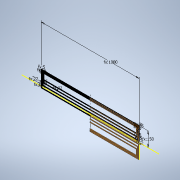
# Autodesk Inventor part: wire_half
Saved by Autodesk Inventor 2020 (Build 240168000, 168)
## iProperties
Created: 2021-01-20
Part Number: wire_half
Material: Generic
Document SubType Name: Modeling
Designer: phamv
Density: 1 g/cm^3
Appearance: Default
Author: phamv
Autodesk Inventor part; units mm, degrees
ref_plane "YZ Plane" through (0, 0, 0) normal (1, 0, 0) x (0, 1, 0)
ref_plane "XY Plane" through (0, 0, 0) normal (0, 0, 1) x (1, 0, 0)
sketch "Sketch1" plane through (0, 0, 0) normal (0, 0, 1) x (1, 0, 0)
  line L0 (0, -11) -> (500, -11)
  line L1 (500, -11) -> (500, -150)
  line L2 (500, -150) -> (-500, -150)
  line L3 (-500, -150) -> (-500, -38)
  line L4 (0, -11) -> (0, -16)
  line L5 (0, -16) -> (495, -16)
  line L6 (495, -16) -> (495, -145)
  line L7 (495, -145) -> (-495, -145)
  line L8 (-500, -38) -> (490, -38)
  line L9 (490, -38) -> (490, -140)
  line L10 (490, -140) -> (-490, -140)
  line L11 (-495, -145) -> (-495, -43)
  line L12 (-495, -43) -> (485, -43)
  line L13 (485, -43) -> (485, -135)
  line L14 (485, -135) -> (-485, -135)
  line L15 (-485, -135) -> (-485, -70)
  line L16 (-490, -140) -> (-490, -65)
  line L17 (-490, -65) -> (480, -65)
  line L18 (480, -65) -> (480, -130)
  line L19 (-485, -70) -> (475, -70)
  line L20 (475, -70) -> (475, -125)
  line L21 (-700, 0) -> (700, 0) projected
  line L22 (475, -125) -> (-480, -125)
  line L23 (480, -130) -> (-480, -130)
  line L24 (-480, -130) -> (-480, -125)
  line L25 (0, -150) -> (0, -11)
  point P0 (0, 0)
  point P1 (0, 0)
  dimension "d1" = 5
  dimension "d2" = 5
  dimension "d3" = 5
  dimension "d4" = 11
  dimension "d5" = 1000
  dimension "d6" = 500
  dimension "d7" = 5
  dimension "d8" = 5
  dimension "d9" = 5
  dimension "d10" = 5
  dimension "d11" = 22
  dimension "d12" = 5
  dimension "d13" = 5
  dimension "d14" = 5
  dimension "d15" = 5
  dimension "d16" = 5
  dimension "d17" = 5
  dimension "d19" = 22
  dimension "d20" = 5
  dimension "d82" = 150
  dimension "d88" = 5
  dimension "d89" = 5
  dimension "d90" = 5
  constraints: 50 end point, 15 perpendicular, 4 horizontal, 3 vertical, 2 parallel, 1 coincident, 1 collinear, 1 midpoint
  measures "d1" distance between parallel lines of L5 L0
  measures "d2" distance between parallel lines of L6 L1
  measures "d3" distance between parallel lines of L2 L7
  measures "d4" distance from line of L21 L0.start
  measures "d5" distance between parallel lines of L3 L1
  measures "d6" distance from line of point (0, 0) L1
  measures "d7" distance between parallel lines of L3 L11
  measures "d8" distance between parallel lines of L13 L9
  measures "d9" distance between parallel lines of L9 L6
  measures "d10" distance between parallel lines of L8 L12
  measures "d11" distance between parallel lines of L8 L5
  measures "d12" distance between parallel lines of L10 L14
  measures "d13" distance between parallel lines of L7 L10
  measures "d14" distance between parallel lines of L16 L15
  measures "d15" distance between parallel lines of L17 L19
  measures "d16" distance between parallel lines of L20 L18
  measures "d17" distance between parallel lines of L18 L13
  measures "d19" distance between parallel lines of L17 L12
  measures "d20" distance between parallel lines of L11 L16
  measures "d82" distance between parallel lines of L2 L21
  measures "d88" distance between parallel lines of L23 L22
  measures "d89" distance between parallel lines of L14 L23
  measures "d90" distance between parallel lines of L15 L24
extrude "Extrusion1" add sketch "Sketch1" along normal blind 5 contours L0 L1 L2 L25 L7 L6 L5 L4 | L25 L12 L11 L7 L2 L3 L8 | L8 L9 L10 L25 L14 L13 L12 | L25 L19 L15 L14 L10 L16 L17 | L17 L18 L23 L25 L22 L20 L19 | L25 L23 L24 L22
sketch "Sketch3" plane through (0, 0, 0) normal (0, 0, 1) x (1, 0, 0)
  line L0 (0, -16) -> (-500, -16)
  line L1 (-500, -16) -> (-500, 150)
  line L2 (-500, 150) -> (500, 150)
  line L3 (500, 150) -> (500, 11)
  line L4 (0, -11) -> (-495, -11)
  line L5 (-495, -11) -> (-495, 145)
  line L6 (-495, 145) -> (495, 145)
  line L7 (495, 145) -> (495, 16)
  line L8 (495, 16) -> (-485, 16)
  line L9 (-485, 16) -> (-485, 135)
  line L10 (500, 11) -> (-490, 11)
  line L11 (-490, 11) -> (-490, 140)
  line L12 (-485, 135) -> (485, 135)
  line L13 (-490, 140) -> (490, 140)
  line L14 (485, 135) -> (485, 43)
  line L15 (485, 43) -> (-475, 43)
  line L16 (490, 140) -> (490, 38)
  line L17 (490, 38) -> (-480, 38)
  line L18 (-475, 43) -> (-475, 125)
  line L19 (-475, 125) -> (475, 125)
  line L20 (475, 125) -> (475, 70)
  line L21 (475, 70) -> (-470, 70)
  line L22 (-480, 38) -> (-480, 130)
  line L23 (-480, 130) -> (480, 130)
  line L24 (480, 130) -> (480, 65)
  line L25 (480, 65) -> (-470, 65)
  line L26 (-470, 70) -> (-470, 65)
  line L27 (500, -150) -> (500, -11) projected
  line L28 (-700, 0) -> (700, 0) projected
  line L29 (0, 150) -> (0, -150) construction
  point P0 (0, 0)
  dimension "d58" = 5
  dimension "d59" = 5
  dimension "d60" = 5
  dimension "d61" = 5
  dimension "d62" = 5
  dimension "d64" = 5
  dimension "d65" = 5
  dimension "d66" = 5
  dimension "d67" = 5
  dimension "d68" = 1000
  dimension "d69" = 22
  dimension "d70" = 5
  dimension "d71" = 5
  dimension "d72" = 22
  dimension "d73" = 5
  dimension "d74" = 5
  dimension "d75" = 5
  dimension "d76" = 5
  dimension "d77" = 22
  dimension "d78" = 5
  dimension "d79" = 5
  dimension "d80" = 5
  dimension "d83" = 150
  dimension "d87" = 5
  constraints: 56 end point, 16 perpendicular, 4 parallel, 4 vertical, 3 horizontal, 1 collinear, 1 midpoint, 1 other
  measures "d58" distance between parallel lines of L1 L5
  measures "d59" distance between parallel lines of L2 L6
  measures "d60" distance between parallel lines of L7 L3
  measures "d61" distance between parallel lines of L13 L6
  measures "d62" distance between parallel lines of L5 L11
  measures "d64" distance between parallel lines of L10 L8
  measures "d65" distance between parallel lines of L14 L16
  measures "d66" distance between parallel lines of L13 L12
  measures "d67" distance between parallel lines of L16 L7
  measures "d68" distance between parallel lines of L1 L3
  measures "d69" distance between parallel lines of L4 L10
  measures "d70" distance between parallel lines of L11 L9
  measures "d71" distance between parallel lines of L17 L15
  measures "d72" distance between parallel lines of L8 L17
  measures "d73" distance between parallel lines of L12 L23
  measures "d74" distance between parallel lines of L9 L22
  measures "d75" distance between parallel lines of L23 L19
  measures "d76" distance between parallel lines of L24 L14
  measures "d77" distance between parallel lines of L15 L25
  measures "d78" distance between parallel lines of L24 L20
  measures "d79" distance between parallel lines of L25 L21
  measures "d80" distance between parallel lines of L22 L18
  measures "d83" distance of the line from the sketch origin of L2
  measures "d87" distance between parallel lines of L18 L26
extrude "Extrusion2" add sketch "Sketch3" along normal blind 5 fills toward (-247.5, -11.05) open curves L4 L5 L6 L7 L8 L9 L12 L14 L15 L18 L19 L20 L21 L26 L25 L24 L23 L22 L17 L16 L13 L11 L10 L3 L2 L1 L0
sketch "Sketch5" plane through (0, 0, 5) normal (0, 0, 1) x (1, 0, 0)
  line L0 (500, 150) -> (-500, 150) projected
  line L1 (-500, -150) -> (500, -150) projected
  line L2 (-500, 150) -> (0, 150)
  line L3 (0, 150) -> (0, -150)
  line L4 (0, -150) -> (-500, -150)
  line L5 (-500, -150) -> (-500, 150)
  point P0 (0, 0)
  constraints: 8 end point, 2 parallel, 1 horizontal, 1 midpoint, 1 perpendicular
extrude "Extrusion3" cut sketch "Sketch5" against normal up to surface (5 mm away)
equation "\"d1\" = wire_diameter"
equation "\"d2\" = wire_diameter"
equation "\"d3\" = wire_diameter"
equation "\"d4\" = 0.5 * distance_between_wires"
equation "\"d5\" = track_length"
equation "\"d6\" = 0.5 * track_length"
equation "\"d7\" = wire_diameter"
equation "\"d8\" = wire_diameter"
equation "\"d9\" = distance_between_wires_edge"
equation "\"d10\" = wire_diameter"
equation "\"d11\" = distance_between_wires"
equation "\"d12\" = wire_diameter"
equation "\"d13\" = distance_between_wires_edge"
equation "\"d14\" = wire_diameter"
equation "\"d15\" = wire_diameter"
equation "\"d16\" = wire_diameter"
equation "\"d17\" = distance_between_wires_edge"
equation "\"d19\" = distance_between_wires"
equation "\"d20\" = distance_between_wires_edge"
equation "\"d82\" = 0.5 * track_width"
equation "\"d22\" = wire_diameter"
equation "\"d58\" = wire_diameter"
equation "\"d59\" = wire_diameter"
equation "\"d60\" = wire_diameter"
equation "\"d61\" = distance_between_wires_edge"
equation "\"d62\" = distance_between_wires_edge"
equation "\"d64\" = wire_diameter"
equation "\"d65\" = wire_diameter"
equation "\"d66\" = wire_diameter"
equation "\"d67\" = distance_between_wires_edge"
equation "\"d68\" = track_length"
equation "\"d69\" = distance_between_wires"
equation "\"d70\" = wire_diameter"
equation "\"d71\" = wire_diameter"
equation "\"d72\" = distance_between_wires"
equation "\"d73\" = distance_between_wires_edge"
equation "\"d74\" = distance_between_wires_edge"
equation "\"d75\" = wire_diameter"
equation "\"d76\" = wire_diameter"
equation "\"d77\" = distance_between_wires"
equation "\"d78\" = wire_diameter"
equation "\"d79\" = wire_diameter"
equation "\"d80\" = wire_diameter"
equation "\"d83\" = 0.5 * track_width"
equation "\"d85\" = wire_diameter"
equation "\"track_length\" = 1000"
equation "\"wire_diameter\" = 5"
equation "\"distance_between_wires\" = -1.2 * wire_diameter + 0.2 * parameter_6"
equation "\"distance_between_wires_edge\" = 5"
equation "\"d53\" = 5"
equation "\"d55\" = 5"
equation "\"d56\" = -1.2 * d53 + 0.2 * d57"
equation "\"d84\" = wire_diameter"
equation "\"track_width\" = 300"
equation "\"parameter_6\" = 140"
equation "\"d57\" = 120"
body "Solid1"
